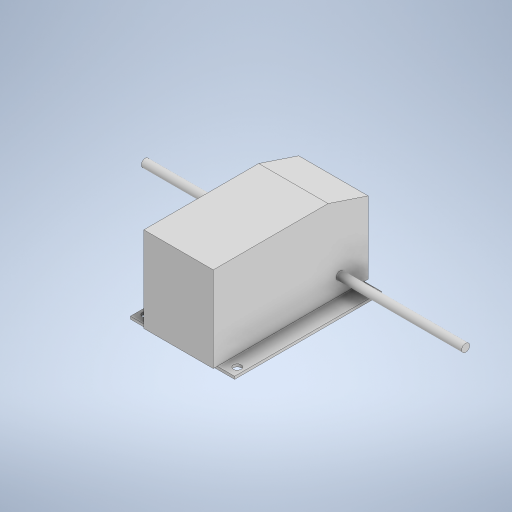
# Autodesk Inventor part: Langbektang houder
Saved by Autodesk Inventor 2023.2 (Build 272271000, 271)
## iProperties
Created: 2020-09-09
Part Number: Langbektang houder
Material: Generic
Document SubType Name: Modeling
Designer: nathan.bollaert
Density: 1 g/cm^3
Appearance: Default
Author: nathan.bollaert
Autodesk Inventor part; units mm, degrees
ref_plane "YZ Plane" through (0, 0, 0) normal (1, 0, 0) x (0, 1, 0)
ref_plane "XZ Plane" through (0, 0, 0) normal (0, 1, 0) x (-1, 0, 0)
sketch "Sketch1" plane through (0, 0, 0) normal (0, 1, 0) x (-1, 0, 0)
  line L0 (0, 0) -> (-39, 0)
  line L1 (-39, 0) -> (-39, -55)
  line L2 (-39, -55) -> (0, -55)
  line L3 (0, -55) -> (0, 0)
  dimension "d228" = 39
  dimension "d229" = 55
  constraints: 8 end point, 2 parallel, 1 coincident, 1 horizontal, 1 perpendicular
  measures "d228" distance of L2.end L1.end
  measures "d229" distance of L1.end L0.end
extrude "Extrusion1" add sketch "Sketch1" along normal blind 1
sketch "Sketch2" plane through (0, 1, 0) normal (0, 1, 0) x (1, 0, 0)
  circle A0 centre (2.5, 3.5) radius 1.5
  circle A1 centre (36.5, 3.5) radius 1.5
  circle A2 centre (2.5, 52) radius 1.5
  circle A3 centre (36.5, 52) radius 1.5
  line L0 (0, 55) -> (0, 0) projected
  line L1 (39, 55) -> (0, 55) projected
  line L2 (39, 0) -> (39, 55) projected
  dimension "d232" = 3
  dimension "d236" = 3.5
  dimension "d237" = 2.5
  dimension "d238" = 3
  dimension "d239" = 2.5
  constraints: 4 centre point, 3 equal radius, 2 horizontal alignment, 2 vertical alignment
  measures "d232" diameter of A0
  measures "d236" vertical distance of L0.end A0.centre
  measures "d237" distance from line of L0 A0.centre
  measures "d238" distance from line of L1 A2.centre
  measures "d239" distance from line of L2 A1.centre
hole "Hole1" at (2.5, 1, -3.5) at (2.5, 1, -52) at (36.5, 1, -52) at (36.5, 1, -3.5) direction (0, -1, 0) diameter 3 end through all
sketch "Sketch3" plane through (0, 1, 0) normal (0, 1, 0) x (1, 0, 0)
  line L0 (0, 0) -> (39, 0) projected
  line L1 (39, 55) -> (0, 55) projected
  line L2 (6.5, 56.5) -> (32.5, 56.5)
  line L3 (32.5, 56.5) -> (32.5, -1.5)
  line L4 (32.5, -1.5) -> (6.5, -1.5)
  line L5 (6.5, -1.5) -> (6.5, 56.5)
  dimension "d257" = 26
  dimension "d258" = 58
  dimension "d259" = 6.5
  dimension "d260" = 1.5
  constraints: 8 end point, 2 parallel, 1 horizontal, 1 perpendicular
  measures "d257" distance of L3.end L4.end
  measures "d258" distance of L2.end L3.end
  measures "d259" horizontal distance of L0.start L4.end
  measures "d260" vertical distance of L0.end L3.end
extrude "Extrusion2" add sketch "Sketch3" along normal blind 32
chamfer "Chamfer1" distance 15 distance2 5 1 edges at (19.5, 33, -56.5) measured on face at (15.1667, 33, -37.1667)
ref_plane "Work Plane" through (19.5, 1, 0) normal (1, 0, 0) x (0, 0, -1)
sketch "Sketch4" plane through (19.5, 1, 0) normal (1, 0, 0) x (0, 0, -1)
  circle A0 centre (46, 6.5) radius 1.5
  line L0 (56.5, 0) -> (56.5, 27) projected
  line L1 (0, 0) -> (55, 0) projected
  point P0 (0, -1)
  dimension "d272" = 3
  dimension "d273" = 10.5
  dimension "d274" = 6.5
  constraints: 1 centre point
  measures "d272" diameter of A0
  measures "d273" distance from line of L0 A0.centre
  measures "d274" distance from line of L1 A0.centre
extrude "Extrusion3" add sketch "Sketch4" along normal mid plane 120
body "Solid5"
